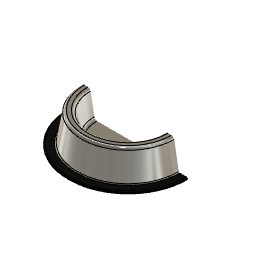
day 11 dog bowl v2 (Autodesk Fusion 360 design; units mm, degrees)
Autodesk Fusion 360 part; units mm, degrees
sketch "Sketch1" plane through (0, 0, 0) normal (0, 1, 0) x (1, 0, 0) in component "dog bowl"
  line L0 (0, 0) -> (110, 0) construction
  line L1 (110, 0) -> (110, -2.5)
  line L2 (110, -2.5) -> (95, -2.5)
  line L3 (95, -2.5) -> (85.4494, -56.6644)
  line L4 (85.4494, -56.6644) -> (70.4494, -56.6644)
  line L5 (70.4494, -56.6644) -> (62.2212, -10)
  line L6 (0, -10) -> (62.2212, -10)
  dimension "d1" = 110
  dimension "d2" = 2.5
  dimension "d3" = 15
  dimension "d4" = 100
  dimension "d5" = 55
  dimension "d6" = 15
  dimension "d7" = 10
  dimension "d8" = 100
  constraint coincident L0.start origin
  constraint horizontal L0
  constraint perpendicular L0 L1
  constraint perpendicular L1 L2
  constraint parallel L2 L4
  constraint horizontal L6
  constraint vertical L0.start L6.start
  measures "d1" distance of L0.start L0.end
  measures "d2" distance of L0.end L1.end
  measures "d3" distance of L1.end L2.end
  measures "d4" angle of L2 L3
  measures "d5" distance of L2.end L3.end
  measures "d6" distance of L3.end L4.end
  measures "d7" distance of L0 L6
  measures "d8" angle of L5 L6
surface "Revolve1" add revolved angle 360 about axis through (0, 0, 1.75) along (0, 0, 20.75) path "Sketch1" along L1 L2 L3 L4 L5 L6 makes body 1 in component "dog bowl"
fillet "Fillet1" radius 5 3 edges at (-79.6668, -30.8998, 56.6644) (-65.6819, -25.4756, 56.6644) (-58.0105, -22.5001, 10) on bodies 1 in component "dog bowl"
fillet "Fillet1" radius 2.5 1 edges at (-88.5711, -34.3535, 2.5) on bodies 1 in component "dog bowl"
thicken "Thicken1" add thickness -2.5 9 faces at (-33.5443, -85.4695, 20.5548) (83.9774, -4.1911, 55.7878) (78.4704, -7.7452, 56.6644) (65.3504, -35.5879, 56.659) (-24.6473, -62.8003, 39.7324) (16.9828, 60.3603, 13.2353) (-30.1138, -10.8957, 10) (95.1609, -4.7493, 3.2844) (104.9282, -10.2888, 2.5) separate body on bodies 1 makes body 2 in component "dog bowl"
fillet "Fillet2" radius 0.5 2 edges at (-102.556, -39.7777, 2.5) (-102.556, -39.7777, 0) on bodies 2 in component "dog bowl"
offset_surface "SurfaceOffset1" offset 0.3 5 faces at (104.9582, -5.44, 0) (87.6312, 66.378, 0.25) (19.1013, -108.3289, 1) (-13.6695, -109.0798, 2.25) (104.9582, -5.44, 2.5) on bodies 2 makes body 3 in component "dog bowl"
thicken "Thicken2" add thickness 1 5 faces at (104.9582, -5.44, 2.8) (50.2711, -98.0575, 2.4) (-29.8737, -106.1775, 1) (87.8383, 66.5349, 0.1) (104.9582, -5.44, -0.3) separate body on bodies 3 makes body 4 in component "dog bowl"
component "dog bowl" placed x (1, 0, 0) y (0, 1, 0) z (0, 0, 1) at (0, 0, 0)
hidden bodies 1 3
